Autodesk Fusion 360 part; units mm, degrees
(part 18 of 18)
  spline S15 degree 5 poles (-4.807101, 4.312986) (-4.8068, 4.310485) (-4.806196, 4.305485) (-4.80528, 4.297995) (-4.804039, 4.288029) (-4.802455, 4.275606) (-4.800837, 4.263216) (-4.799187, 4.250862) (-4.797505, 4.238541) (-4.795789, 4.226254) (-4.794041, 4.214003) (-4.792261, 4.201786) (-4.790449, 4.189603) (-4.788604, 4.177456) (-4.786728, 4.165345) (-4.78482, 4.153268) (-4.782881, 4.141228) (-4.780911, 4.129223) (-4.77891, 4.117255) (-4.776878, 4.105322) (-4.774815, 4.093426) (-4.772721, 4.081567) (-4.770598, 4.069744) (-4.768444, 4.057958) (-4.76626, 4.046208) (-4.764046, 4.034497) (-4.761803, 4.022822) (-4.75953, 4.011185) (-4.757228, 3.999586) (-4.754896, 3.988024) (-4.752536, 3.976501) (-4.750148, 3.965016) (-4.74773, 3.953569) (-4.745285, 3.942161) (-4.742811, 3.930791) (-4.740309, 3.919461) (-4.73778, 3.908169) (-4.735223, 3.896917) (-4.732638, 3.885704) (-4.730027, 3.87453) (-4.727389, 3.863396) (-4.724723, 3.852302) (-4.722032, 3.841249) (-4.719314, 3.830235) (-4.716569, 3.819262) (-4.713799, 3.808329) (-4.711004, 3.797437) (-4.708182, 3.786586) (-4.705336, 3.775776) (-4.702464, 3.765007) (-4.699568, 3.75428) (-4.696647, 3.743594) (-4.693701, 3.732949) (-4.690731, 3.722347) (-4.687737, 3.711787) (-4.68472, 3.701269) (-4.681679, 3.690793) (-4.678615, 3.68036) (-4.675527, 3.669969) (-4.672417, 3.659621) (-4.669284, 3.649317) (-4.666129, 3.639055) (-4.662952, 3.628837) (-4.659752, 3.618662) (-4.656532, 3.608531) (-4.653289, 3.598444) (-4.650026, 3.588401) (-4.646741, 3.578402) (-4.643436, 3.568447) (-4.64011, 3.558537) (-4.636764, 3.548671) (-4.633399, 3.538851) (-4.630013, 3.529075) (-4.626608, 3.519344) (-4.623184, 3.509659) (-4.619741, 3.500019) (-4.616279, 3.490424) (-4.612799, 3.480876) (-4.609301, 3.471373) (-4.605784, 3.461916) (-4.602251, 3.452506) (-4.598699, 3.443142) (-4.595131, 3.433824) (-4.591546, 3.424554) (-4.587945, 3.41533) (-4.584327, 3.406153) (-4.580693, 3.397023) (-4.577043, 3.387941) (-4.573378, 3.378906) (-4.569698, 3.369918) (-4.566003, 3.360979) (-4.562294, 3.352087) (-4.55857, 3.343244) (-4.554832, 3.334449) (-4.551081, 3.325702) (-4.547316, 3.317004) (-4.543538, 3.308354) (-4.539748, 3.299753) (-4.535945, 3.291202) (-4.532129, 3.282699) (-4.528302, 3.274246) (-4.524464, 3.265842) (-4.520614, 3.257488) (-4.516753, 3.249184) (-4.512882, 3.24093) (-4.509, 3.232725) (-4.505108, 3.224571) (-4.501207, 3.216468) (-4.497297, 3.208415) (-4.493377, 3.200412) (-4.489449, 3.19246) (-4.485512, 3.184559) (-4.481568, 3.17671) (-4.477616, 3.168911) (-4.473657, 3.161164) (-4.469691, 3.153469) (-4.465718, 3.145825) (-4.461739, 3.138233) (-4.457754, 3.130693) (-4.453764, 3.123205) (-4.449768, 3.11577) (-4.445768, 3.108386) (-4.441763, 3.101056) (-4.437754, 3.093777) (-4.433742, 3.086552) (-4.429726, 3.07938) (-4.425707, 3.072261) (-4.421686, 3.065195) (-4.417663, 3.058182) (-4.413637, 3.051223) (-4.409611, 3.044318) (-4.405583, 3.037466) (-4.401555, 3.030668) (-4.397527, 3.023924) (-4.393499, 3.017235) (-4.389471, 3.0106) (-4.385445, 3.004019) (-4.38142, 2.997493) (-4.377397, 2.991021) (-4.373376, 2.984604) (-4.369358, 2.978243) (-4.365343, 2.971936) (-4.361331, 2.965685) (-4.357324, 2.959489) (-4.353321, 2.953348) (-4.349323, 2.947263) (-4.34533, 2.941234) (-4.341344, 2.935261) (-4.337363, 2.929344) (-4.333389, 2.923482) (-4.329422, 2.917678) (-4.325463, 2.911929) (-4.321513, 2.906237) (-4.31757, 2.900601) (-4.313637, 2.895022) (-4.309713, 2.8895) (-4.3058, 2.884035) (-4.301897, 2.878627) (-4.298005, 2.873277) (-4.294125, 2.867983) (-4.290256, 2.862747) (-4.286401, 2.857569) (-4.282558, 2.852448) (-4.278729, 2.847385) (-4.274915, 2.842379) (-4.271115, 2.837432) (-4.26733, 2.832543) (-4.263561, 2.827712) (-4.259809, 2.822939) (-4.256073, 2.818225) (-4.252355, 2.813569) (-4.248655, 2.808972) (-4.244974, 2.804434) (-4.241312, 2.799954) (-4.237669, 2.795533) (-4.234047, 2.791172) (-4.230446, 2.786869) (-4.226867, 2.782626) (-4.22331, 2.778442) (-4.219776, 2.774317) (-4.216265, 2.770252) (-4.212779, 2.766246) (-4.209317, 2.762301) (-4.20588, 2.758415) (-4.20247, 2.754588) (-4.199087, 2.750822) (-4.19573, 2.747116) (-4.192402, 2.74347) (-4.189103, 2.739884) (-4.185834, 2.736358) (-4.182594, 2.732893) (-4.179385, 2.729488) (-4.176209, 2.726144) (-4.173064, 2.72286) (-4.169953, 2.719637) (-4.166875, 2.716475) (-4.163832, 2.713374) (-4.160825, 2.710333) (-4.157854, 2.707354) (-4.154919, 2.704435) (-4.152023, 2.701577) (-4.149165, 2.698781) (-4.146347, 2.696046) (-4.143569, 2.693372) (-4.140832, 2.69076) (-4.138137, 2.688209) (-4.135485, 2.685719) (-4.132877, 2.683291) (-4.130313, 2.680924) (-4.127795, 2.678619) (-4.125323, 2.676376) (-4.122899, 2.674194) (-4.120524, 2.672074) (-4.118197, 2.670016) (-4.115921, 2.66802) (-4.113697, 2.666085) (-4.111524, 2.664213) (-4.109406, 2.662402) (-4.107341, 2.660653) (-4.105333, 2.658966) (-4.10338, 2.657341) (-4.101486, 2.655778) (-4.09965, 2.654277) (-4.097875, 2.652839) (-4.09616, 2.651462) (-4.094508, 2.650147) (-4.09292, 2.648895) (-4.091396, 2.647704) (-4.089938, 2.646575) (-4.088548, 2.645509) (-4.087226, 2.644505) (-4.085975, 2.643562) (-4.084794, 2.642682) (-4.083687, 2.641864) (-4.082653, 2.641108) (-4.081694, 2.640414) (-4.080812, 2.639782) (-4.080009, 2.639211) (-4.079287, 2.638703) (-4.078647, 2.638256) (-4.078091, 2.637872) (-4.077713, 2.637613) (-4.077467, 2.637448) (-4.07732, 2.637349) (-4.077251, 2.637303) knots -1 -1 -1 -1 -1 -1 -0.99583333 -0.99166667 -0.9875 -0.98333333 -0.97916667 -0.975 -0.97083333 -0.96666667 -0.9625 -0.95833333 -0.95416667 -0.95 -0.94583333 -0.94166667 -0.9375 -0.93333333 -0.92916667 -0.925 -0.92083333 -0.91666667 -0.9125 -0.90833333 -0.90416667 -0.9 -0.89583333 -0.89166667 -0.8875 -0.88333333 -0.87916667 -0.875 -0.87083333 -0.86666667 -0.8625 -0.85833333 -0.85416667 -0.85 -0.84583333 -0.84166667 -0.8375 -0.83333333 -0.82916667 -0.825 -0.82083333 -0.81666667 -0.8125 -0.80833333 -0.80416667 -0.8 -0.79583333 -0.79166667 -0.7875 -0.78333333 -0.77916667 -0.775 -0.77083333 -0.76666667 -0.7625 -0.75833333 -0.75416667 -0.75 -0.74583333 -0.74166667 -0.7375 -0.73333333 -0.72916667 -0.725 -0.72083333 -0.71666667 -0.7125 -0.70833333 -0.70416667 -0.7 -0.69583333 -0.69166667 -0.6875 -0.68333333 -0.67916667 -0.675 -0.67083333 -0.66666667 -0.6625 -0.65833333 -0.65416667 -0.65 -0.64583333 -0.64166667 -0.6375 -0.63333333 -0.62916667 -0.625 -0.62083333 -0.61666667 -0.6125 -0.60833333 -0.60416667 -0.6 -0.59583333 -0.59166667 -0.5875 -0.58333333 -0.57916667 -0.575 -0.57083333 -0.56666667 -0.5625 -0.55833333 -0.55416667 -0.55 -0.54583333 -0.54166667 -0.5375 -0.53333333 -0.52916667 -0.525 -0.52083333 -0.51666667 -0.5125 -0.50833333 -0.50416667 -0.5 -0.49583333 -0.49166667 -0.4875 -0.48333333 -0.47916667 -0.475 -0.47083333 -0.46666667 -0.4625 -0.45833333 -0.45416667 -0.45 -0.44583333 -0.44166667 -0.4375 -0.43333333 -0.42916667 -0.425 -0.42083333 -0.41666667 -0.4125 -0.40833333 -0.40416667 -0.4 -0.39583333 -0.39166667 -0.3875 -0.38333333 -0.37916667 -0.375 -0.37083333 -0.36666667 -0.3625 -0.35833333 -0.35416667 -0.35 -0.34583333 -0.34166667 -0.3375 -0.33333333 -0.32916667 -0.325 -0.32083333 -0.31666667 -0.3125 -0.30833333 -0.30416667 -0.3 -0.29583333 -0.29166667 -0.2875 -0.28333333 -0.27916667 -0.275 -0.27083333 -0.26666667 -0.2625 -0.25833333 -0.25416667 -0.25 -0.24583333 -0.24166667 -0.2375 -0.23333333 -0.22916667 -0.225 -0.22083333 -0.21666667 -0.2125 -0.20833333 -0.20416667 -0.2 -0.19583333 -0.19166667 -0.1875 -0.18333333 -0.17916667 -0.175 -0.17083333 -0.16666667 -0.1625 -0.15833333 -0.15416667 -0.15 -0.14583333 -0.14166667 -0.1375 -0.13333333 -0.12916667 -0.125 -0.12083333 -0.11666667 -0.1125 -0.10833333 -0.10416667 -0.1 -0.09583333 -0.09166667 -0.0875 -0.08333333 -0.07916667 -0.075 -0.07083333 -0.06666667 -0.0625 -0.05833333 -0.05416667 -0.05 -0.04583333 -0.04166667 -0.0375 -0.03333333 -0.02916667 -0.025 -0.02083333 -0.01666667 -0.0125 -0.00833333 -0.00416667 0 0 0 0 0 0
  line L30 (-4.077251, 2.637303) -> (-4.076603, 2.636873)
  line L31 (-4.076603, 2.636873) -> (-2.982533, 1.929195)
  circle A16 centre (0, 0) radius 2.975
  line L32 (3, 1) -> (-3, 1)
  line L33 (-3, 1) -> (-3, -1)
  line L34 (-3, -1) -> (3, -1)
  line L35 (3, -1) -> (3, 1)
  line L36 (3, 1) -> (-3, -1) construction
  line L37 (-3, 1) -> (3, -1) construction
  line L38 (0, -1) -> (0, 1)
  line L39 (0.1, -1) -> (0.1, 1)
  line L40 (2.899688, -0.899688) -> (2.899688, 0.899688)
  line L41 (2.899688, 0.899688) -> (-2.899688, 0.899688)
  line L42 (-2.899688, 0.899688) -> (-2.899688, -0.899688)
  line L43 (-2.899688, -0.899688) -> (2.899688, -0.899688)
  dimension "d13" = 5.95
  dimension "d14" = 6
  dimension "d15" = 2
  dimension "d16" = -0.100312
  constraint coincident A0.centre A1.centre
  constraint horizontal L32
  constraint perpendicular L32 L33
  constraint parallel L32 L34
  constraint parallel L33 L35
  constraint coincident L36 A0.centre
  constraint coincident L37 A0.centre
  constraint midpoint L34 L38.start
  constraint midpoint L32 L38.end
  constraint coincident L34 L39.start
  constraint coincident L32 L39.end
  constraint perpendicular L32 L39
  measures "d13" diameter of A16
  measures "d14" distance of L33.end L34.end
  measures "d15" distance of L32.end L33.end
extrude "Extrude3" cut sketch "Sketch1 (3)" against normal blind 3 contours A16 L32 L39 L41 | A16 L34 L39 L43 | A16 L32 | L32 L38 L39 L41 | L38 L39 L41 L43 | A16 L34 | L34 L38 L39 L43 | A16 L32 L38 L41 | A16 L38 L41 L42 L43 | A16 L34 L38 L43 | A16 L42 picked at (1.000632, 0.966563) picked at (1.000632, -0.966563) picked at (0, 2.311495) picked at (0.066667, 0.933125) picked at (0.033333, 0.299896) picked at (0, -2.311495) picked at (0.033333, -0.933125) picked at (-0.933966, 0.966563) picked at (-0.966563, 0.221719) picked at (-0.933966, -0.966563) picked at (-2.918496, 0.111568) bodies 1 in component "Component"
extrude "Extrude3'" cut sketch "Sketch1 (3)" against normal blind 3 contours A16 L32 L39 L41 | A16 L34 L39 L43 | A16 L32 | L32 L38 L39 L41 | L38 L39 L41 L43 | A16 L34 | L34 L38 L39 L43 | A16 L32 L38 L41 | A16 L38 L41 L42 L43 | A16 L34 L38 L43 | A16 L42 picked at (1.000632, 0.966563) picked at (1.000632, -0.966563) picked at (0, 2.311495) picked at (0.066667, 0.933125) picked at (0.033333, 0.299896) picked at (0, -2.311495) picked at (0.033333, -0.933125) picked at (-0.933966, 0.966563) picked at (-0.966563, 0.221719) picked at (-0.933966, -0.966563) picked at (-2.918496, 0.111568) bodies 10 in component "Component'"
extrude "Extrude4" add 1 faces at (-1.923799, 0.299896, 3) along direction (0, 0, 1) blind 2 on bodies 1 bodies 1 in component "Component"
component "Component'" placed x (1, 0, 0) y (0, 1, 0) z (0, 0, 1) at (21, 0, 0)
component "Component" placed x (1, 0, 0) y (0, 1, 0) z (0, 0, 1) at (0, 0, 0)
